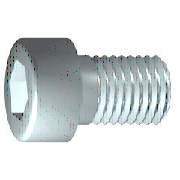
# Autodesk Inventor part: M3 x 5 - Socket Cap Screw - Standard (A2)
Saved by Autodesk Inventor 2016 SP1 (Build 200210100, 210)
## iProperties
Created: 2017-05-23
Part Number: M3 x 5 - Socket Cap Screw - Standard (A2)
Cost Center: P
Material: Stainless Steel
Description: Socket Cap Screw - Standard - (A2) - M3 x 5
Vendor: Generic Manufacturer
Document SubType Name: Modeling
Standard: ISO 4762
Designer: Matthew Lockham
Standard Revision: Fourth edition 2004-03-01
Standards Organization: ISO
Language: en-US
Size Designation: M3 x 5
Categories: <MemberInstance><Categories><Category DisplayName="Fasteners" InternalName="e4da775c-781d-43d5-af7c-5136215cf5a6" Mnemonic="FSTN"><Category DisplayName="Bolts" InternalName="536e6df0-f778-49ac-b2f2-25c71d2aa0b2" Mnemonic="SCRW"><CategoryParameter DisplayName="Nominal Diameter" InternalName="8bbe3f8e-44cf-40a9-a251-3a6edc8168d6" Mnemonic="nomdia"/><CategoryParameter DisplayName="Nominal Length" InternalName="238ecbaf-3e6c-45dd-aa95-4068c8e0fd02" Mnemonic="nomlen"/><CategoryParameter DisplayName="Thread Series Designation" InternalName="87c5849c-b3a5-4c3e-9c9b-2feecef9be86" Mnemonic="thrserdsgn"/><CategoryParameter DisplayName="Thread Class" InternalName="ebc0d23b-2cc6-4d2a-b376-d52aae53bab6" Mnemonic="thrclss"/><CategoryParameter DisplayName="Thread Designation" InternalName="586d5e89-370a-4089-914f-0110033585c7" Mnemonic="thrdesign"/><CategoryParameter DisplayName="Thread Type" InternalName="b4bbb7bc-d6aa-4c9f-a9a9-4152b9f6fe49" Mnemonic="thrtype"/><CategoryParameter DisplayName="Threads per Unit" InternalName="bdc6e7d2-ffd0-4d9c-a173-16b95ebb912d" Mnemonic="thrperunit1"/><CategoryParameter DisplayName="Thread Pitch" InternalName="bb82302e-82d8-4176-8fc1-c5d7bb17d5ad" Mnemonic="pitch1"/><CategoryParameter DisplayName="Nominal Diameter Designation" InternalName="03caf894-eafd-4c09-a035-916ac084b87b" Mnemonic="nomdiadesig"/><Category DisplayName="Socket Head" InternalName="55e06bf3-7e58-486c-bbdc-745fcc60664d" Mnemonic="CLSCRW"><CategoryParameter DisplayName="Shank Diameter" InternalName="179dbae3-102f-48bb-85fe-1e3ecd34f7cc" Mnemonic="grpdia"/><CategoryParameter DisplayName="Grip Length" InternalName="52eab69f-422f-4795-9995-175a1b827e67" Mnemonic="grplen"/><CategoryParameter DisplayName="Thread Length" InternalName="3268731d-5f9a-4750-8b01-4a959c46fbf2" Mnemonic="thrlen"/><CategoryParameter DisplayName="Head Diameter" InternalName="46177176-dbdd-4a1b-aefd-4c60c45016af" Mnemonic="headdia"/><CategoryParameter DisplayName="Head Height" InternalName="99c92c4c-4a02-4ebe-9e64-948fb169e19e" Mnemonic="headh"/><CategoryParameter DisplayName="Type" InternalName="59a7e495-7a0c-4a5c-bdfd-c090c5f6e2db" Mnemonic="type"/></Category></Category></Category><Category DisplayName="DataType" InternalName="23b78d0f-2648-40c6-8793-ca6db495c9e8" Mnemonic="DATATYPE"><CategoryParameter DisplayName="DisplayName" InternalName="05415f3d-3907-474b-a020-eb9d644f4cf3" Mnemonic="DISPLAYNAME"/><CategoryParameter DisplayName="InternalName" InternalName="cf1d0246-76d9-4b4a-8305-fa0409afb5c1" Mnemonic="INTERNALNAME"/><CategoryParameter DisplayName="Folder Name" InternalName="3f06958e-8713-4116-9be7-ed6184ecc97b" Mnemonic="FOLDERNAME"/><CategoryParameter DisplayName="Family Version" InternalName="914462f6-6e19-4b14-ba84-155b9680b1d0" Mnemonic="FAMILYREVISION"/><CategoryParameter DisplayName="ClipFormat" InternalName="bc51e27b-3422-4e78-93ef-cec197ddf230" Mnemonic="CLIPFORMAT"/><CategoryParameter DisplayName="IsMetric" InternalName="e2385c5b-1ea4-4823-96a8-8de651266ec3" Mnemonic="ISMETRIC"/><CategoryParameter DisplayName="Description" InternalName="13903e3d-64b1-4950-80da-f627842ea37f" Mnemonic="DESCRIPTION"/><CategoryParameter DisplayName="StdsOrg" InternalName="8f5914e1-4693-403f-8ab5-d37768198c9d" Mnemonic="STDSORG"/><CategoryParameter DisplayName="Standard" InternalName="0c0a119c-1e12-4c84-803f-101930972f5e" Mnemonic="STANDARD"/><CategoryParameter DisplayName="Manufacturer" InternalName="cd6c7a72-a28a-4e50-99a9-2c7f4e13e5ad" Mnemonic="MANUFACTURER"/><CategoryParameter DisplayName="Member Revision" InternalName="a65d44b9-392f-4f4f-857b-e4b3d54996fe" Mnemonic="MEMBERREVISION"/><CategoryParameter DisplayName="Standard Revision" InternalName="91d5a463-65c2-4fde-b823-3b7fea5e8e17" Mnemonic="STANDARDREVISION"/><CategoryParameter DisplayName="Revision Guid" InternalName="45a75005-10b1-4dfc-8d6d-dfe629f0b93c" Mnemonic="REVISIONGUID"/><CategoryParameter DisplayName="Designation" InternalName="2675968c-4ce5-49e0-a4f5-552d29089031" Mnemonic="DESIGNATION"/><CategoryParameter DisplayName="FileName" InternalName="8b46a4cc-9585-4fed-90c3-899f57e09a73" Mnemonic="FILENAME"/><CategoryParameter DisplayName="Default Row" InternalName="2af9ec52-faaa-4026-b378-f9fa4afca842" Mnemonic="DEFAULTROW"/><Category DisplayName="Part" InternalName="c0e0b642-3bcb-4cc8-9e80-f96d35c4afa4" Mnemonic="PART"><CategoryParameter DisplayName="Material" InternalName="818a152a-d3c3-49ca-80ee-df7d91421b8e" Mnemonic="MATERIAL"/><CategoryParameter DisplayName="Material Key" InternalName="5c9a8adb-dd2b-4535-b97f-0a94a95fe41f" Mnemonic="MATERIALKEY"/><CategoryParameter DisplayName="Part Number" InternalName="016b6077-bfbe-49bd-92c9-d8d59c39c941" Mnemonic="PARTNUMBER"/><CategoryParameter DisplayName="Stock Number" InternalName="4dba7c1c-e26c-444e-836c-b08b433409a8" Mnemonic="STOCKNUMBER"/></Category></Category></Categories><FamilyTemplate Id="si0145"><FamilyTemplateParameters><FamilyTemplateParameter ObjectType="kUserParameterObject" ValueType="xs:double" Id="1" ObjectReferenceKey="GUL"/><FamilyTemplateParameter ObjectType="kUserParameterObject" ValueType="xs:double" Id="2" ObjectReferenceKey="SPD"/><FamilyTemplateParameter ObjectType="kUserParameterObject" ValueType="xs:double" Id="3" ObjectReferenceKey="NLG"/><FamilyTemplateParameter ObjectType="kUserParameterObject" ValueType="xs:double" Id="4" ObjectReferenceKey="KOD"/><FamilyTemplateParameter ObjectType="kUserParameterObject" ValueType="xs:double" Id="5" ObjectReferenceKey="TOA"/><FamilyTemplateParameter ObjectType="kUserParameterObject" ValueType="xs:double" Id="6" ObjectReferenceKey="GD1"/><FamilyTemplateParameter ObjectType="kUserParameterObject" ValueType="xs:double" Id="7" ObjectReferenceKey="GEL"/><FamilyTemplateParameter ObjectType="kUserParameterObject" ValueType="xs:double" Id="8" ObjectReferenceKey="SW"/><FamilyTemplateParameter ObjectType="kUserParameterObject" ValueType="xs:double" Id="9" ObjectReferenceKey="THREADDIA"/><FamilyTemplateParameter ObjectType="kUserParameterObject" ValueType="xs:double" Id="10" ObjectReferenceKey="INTI"/><FamilyTemplateParameter ObjectType="kUserParameterObject" ValueType="xs:double" Id="11" ObjectReferenceKey="BDM"/><FamilyTemplateParameter ObjectType="kUserParameterObject" ValueType="xs:double" Id="12" ObjectReferenceKey="FAWI"/><FamilyTemplateParameter ObjectType="kUserParameterObject" ValueType="xs:double" Id="13" ObjectReferenceKey="RR"/><FamilyTemplateParameter ObjectType="kUserParameterObject" ValueType="xs:double" Id="14" ObjectReferenceKey="KOH"/><FamilyTemplateParameter ObjectType="kUserParameterObject" ValueType="xs:double" Id="15" ObjectReferenceKey="TPU"/><FamilyTemplateParameter ObjectType="kUserParameterObject" ValueType="xs:double" Id="16" ObjectReferenceKey="PTC"/><FamilyTemplateParameter ObjectType="kUserParameterObject" ValueType="xs:double" Id="17" ObjectReferenceKey="NND"/><FamilyTemplateParameter ObjectType="kUserParameterObject" ValueType="xs:double" Id="18" ObjectReferenceKey="GD"/><FamilyTemplateParameter ObjectType="kUserParameterObject" ValueType="xs:double" Id="19" ObjectReferenceKey="GAL"/><FamilyTemplateParameter ObjectType="kUserParameterObject" ValueType="xs:double" Id="20" ObjectReferenceKey="E0"/><FamilyTemplateParameter ObjectType="kPropertyObject" ValueType="xs:string" Id="100" ObjectReferenceKey="{32853F0F-3444-11d1-9E93-0060B03C1CA6}" SubObjectId="52"/><FamilyTemplateParameter ObjectType="kPropertyObject" ValueType="xs:string" Id="105" ObjectReferenceKey="{32853F0F-3444-11d1-9E93-0060B03C1CA6}" SubObjectId="5"/><FamilyTemplateParameter ObjectType="kPropertyObject" ValueType="xs:string" Id="106" ObjectReferenceKey="{32853F0F-3444-11d1-9E93-0060B03C1CA6}" SubObjectId="29"/><FamilyTemplateParameter ObjectType="kPartComponentDefinitionObject" ValueType="xs:string" Id="110" SubObjectId="Material"/><FamilyTemplateParameter ObjectType="kThreadFeatureObject" ValueType="xs:structure" Id="300" ObjectReferenceKey="1002000010000000a2070000000000008000000000000000" SubObjectId="ThreadInfo"><FamilyTemplateParameter ObjectType="" ValueType="xs:string" Id="301" SubObjectId="ThreadDesignation"/><FamilyTemplateParameter ObjectType="" ValueType="xs:string" Id="302" SubObjectId="ThreadType"/><FamilyTemplateParameter ObjectType="" ValueType="xs:string" Id="303" SubObjectId="ThreadClass"/></FamilyTemplateParameter><FamilyTemplateParameter ObjectType="kPropertyObject" ValueType="xs:string" Id="503" ObjectReferenceKey="{32853F0F-3444-11D1-9E93-0060B03C1CA6}" SubObjectId="9"/><FamilyTemplateParameter ObjectType="kPropertyObject" ValueType="xs:string" Id="504" ObjectReferenceKey="{32853F0F-3444-11D1-9E93-0060B03C1CA6}" SubObjectId="30"/><FamilyTemplateParameter ObjectType="kPartDocumentObject" ValueType="xs:string" Id="505" SubObjectId="DisplayName"/></FamilyTemplateParameters></FamilyTemplate><CategoryParameterMap><ParamToTemplateMap><ParamToTemplate CategoryParameter="//CategoryParameter[@InternalName='05415f3d-3907-474b-a020-eb9d644f4cf3']" ConstantValue="Socket Cap Screw"/><ParamToTemplate CategoryParameter="//CategoryParameter[@InternalName='cf1d0246-76d9-4b4a-8305-fa0409afb5c1']" ConstantValue="0228a834-b69c-46de-845a-346444175acc"/><ParamToTemplate CategoryParameter="//CategoryParameter[@InternalName='3f06958e-8713-4116-9be7-ed6184ecc97b']" ConstantValue="Socket Cap Screw"/><ParamToTemplate CategoryParameter="//CategoryParameter[@InternalName='914462f6-6e19-4b14-ba84-155b9680b1d0']" ConstantValue="10"/><ParamToTemplate CategoryParameter="//CategoryParameter[@InternalName='bc51e27b-3422-4e78-93ef-cec197ddf230']" ConstantValue="CF_INVENTOR.STDPARTS"/><ParamToTemplate CategoryParameter="//CategoryParameter[@InternalName='e2385c5b-1ea4-4823-96a8-8de651266ec3']" ConstantValue="true"/><ParamToTemplate CategoryParameter="//CategoryParameter[@InternalName='13903e3d-64b1-4950-80da-f627842ea37f']" ConstantValue="Hexagon Socket Head Cap Screw"/><ParamToTemplate CategoryParameter="//CategoryParameter[@InternalName='8f5914e1-4693-403f-8ab5-d37768198c9d']" ConstantValue="ISO"/><ParamToTemplate CategoryParameter="//CategoryParameter[@InternalName='0c0a119c-1e12-4c84-803f-101930972f5e']" ConstantValue="ISO 4762"/><ParamToTemplate CategoryParameter="//CategoryParameter[@InternalName='cd6c7a72-a28a-4e50-99a9-2c7f4e13e5ad']" TemplateParameter="104"/><ParamToTemplate CategoryParameter="//CategoryParameter[@InternalName='91d5a463-65c2-4fde-b823-3b7fea5e8e17']" ConstantValue="Fourth edition 2004-03-01"/><ParamToTemplate CategoryParameter="//CategoryParameter[@InternalName='45a75005-10b1-4dfc-8d6d-dfe629f0b93c']" ConstantValue="8a618e3f-b604-4408-b898-144709662ae0"/><ParamToTemplate CategoryParameter="//CategoryParameter[@InternalName='2af9ec52-faaa-4026-b378-f9fa4afca842']" ConstantValue="10"/><ParamToTemplate CategoryParameter="//CategoryParameter[@InternalName='a65d44b9-392f-4f4f-857b-e4b3d54996fe']" ConstantValue="69ce6232-463b-47b9-b677-461f109c7dae"/><ParamToTemplate CategoryParameter="//CategoryParameter[@InternalName='52eab69f-422f-4795-9995-175a1b827e67']" ConstantValue="1.25"/><ParamToTemplate CategoryParameter="//CategoryParameter[@InternalName='ebc0d23b-2cc6-4d2a-b376-d52aae53bab6']" ConstantValue="6g"/><ParamToTemplate CategoryParameter="//CategoryParameter[@InternalName='03caf894-eafd-4c09-a035-916ac084b87b']" ConstantValue="M3"/><ParamToTemplate CategoryParameter="//CategoryParameter[@InternalName='b4bbb7bc-d6aa-4c9f-a9a9-4152b9f6fe49']" ConstantValue="ISO Metric profile"/><ParamToTemplate CategoryParameter="//CategoryParameter[@InternalName='179dbae3-102f-48bb-85fe-1e3ecd34f7cc']" TemplateParameter="11"/><ParamToTemplate CategoryParameter="//CategoryParameter[@InternalName='2675968c-4ce5-49e0-a4f5-552d29089031']" TemplateParameter="100"/><ParamToTemplate CategoryParameter="//CategoryParameter[@InternalName='8b46a4cc-9585-4fed-90c3-899f57e09a73']" TemplateParameter="505"/><ParamToTemplate CategoryParameter="//CategoryParameter[@InternalName='3268731d-5f9a-4750-8b01-4a959c46fbf2']" TemplateParameter="7"/><ParamToTemplate CategoryParameter="//CategoryParameter[@InternalName='46177176-dbdd-4a1b-aefd-4c60c45016af']" TemplateParameter="4"/><ParamToTemplate CategoryParameter="//CategoryParameter[@InternalName='99c92c4c-4a02-4ebe-9e64-948fb169e19e']" TemplateParameter="14"/><ParamToTemplate CategoryParameter="//CategoryParameter[@InternalName='818a152a-d3c3-49ca-80ee-df7d91421b8e']" TemplateParameter="110"/><ParamToTemplate CategoryParameter="//CategoryParameter[@InternalName='238ecbaf-3e6c-45dd-aa95-4068c8e0fd02']" TemplateParameter="3"/><ParamToTemplate CategoryParameter="//CategoryParameter[@InternalName='8bbe3f8e-44cf-40a9-a251-3a6edc8168d6']" TemplateParameter="17"/><ParamToTemplate CategoryParameter="//CategoryParameter[@InternalName='016b6077-bfbe-49bd-92c9-d8d59c39c941']" TemplateParameter="105"/><ParamToTemplate CategoryParameter="//CategoryParameter[@InternalName='bb82302e-82d8-4176-8fc1-c5d7bb17d5ad']" TemplateParameter="16"/><ParamToTemplate CategoryParameter="//CategoryParameter[@InternalName='586d5e89-370a-4089-914f-0110033585c7']" TemplateParameter="301"/><ParamToTemplate CategoryParameter="//CategoryParameter[@InternalName='bdc6e7d2-ffd0-4d9c-a173-16b95ebb912d']" TemplateParameter="15"/></ParamToTemplateMap></CategoryParameterMap></MemberInstance>
Density: 8.08 g/cm^3
Appearance: Metal-Steel (Stainless, Brushed)
Saved_Yet: Not Saved
IsCustomPart: 0
Author: Matthew Lockham
Autodesk Inventor part; units mm, degrees
ref_plane "YZ Plane" through (0, 0, 0) normal (1, 0, 0) x (0, 1, 0)
ref_plane "XZ Plane" through (0, 0, 0) normal (0, 1, 0) x (-1, 0, 0)
ref_plane "XY Plane" through (0, 0, 0) normal (0, 0, 1) x (1, 0, 0)
sketch "Sketch1" plane through (0, 0, 0) normal (0, 0, 1) x (1, 0, 0)
  line L0 (-0.8667, 0) -> (5, 0)
  line L1 (5, 0) -> (5, 1.5)
  line L2 (5, 1.5) -> (1.25, 1.5)
  line L3 (1.25, 1.5) -> (0.9432, 1.5)
  line L4 (0.9432, 1.5) -> (0, 1.5)
  line L5 (0, 1.5) -> (0, 2.75)
  line L6 (0, 2.75) -> (-3, 2.75)
  line L7 (-3, 2.75) -> (-3, 1.4434)
  line L8 (-3, 1.4434) -> (-1.7, 1.4434)
  line L9 (-1.7, 1.4434) -> (-0.8667, 0)
  line L10 (-4.6, 0) -> (6.6, 0) projected
  line L11 (0, -0.55) -> (0, 3.3) projected
  line L12 (1.25, 1.5) -> (0, 1.5) construction
  dimension "d1" = 3.75
  dimension "d2" = 0.3068
  dimension "d3" = 3
  dimension "d4" = 1.3
  dimension "d5" = 60
  dimension "d6" = 3
  dimension "d7" = 3
  dimension "d8" = 2.8868
  dimension "d9" = 5.5
  dimension "d26" = 5
  constraints: 22 end point, 6 parallel, 2 collinear, 2 perpendicular, 1 horizontal, 1 point on line
  measures "d1" distance from line of L2.end L1
  measures "d2" distance of L3.end L2.end
  measures "d3" distance between parallel lines of L7 L5
  measures "d4" distance of L7.end L8.end
  measures "d5" angle of L9 L0
  measures "d6" diameter of L2 L0
  measures "d7" diameter of L4 L0
  measures "d8" diameter of L8 L0
  measures "d9" diameter of L6 L0
  measures "d26" distance between parallel lines of L11 L1
revolve "Body" add sketch "Sketch1" angle 360 about axis through (-0.8667, 0, 0) along (1, 0, 0)
sketch "Sketch2" plane through (-3, 0, 0) normal (-1, 0, 0) x (0, 0, 1)
  circle A0 centre (0, 0) radius 1.4434 projected
  line L0 (0, -3.85) -> (0, 3.85) projected
  line L1 (-3.85, 0) -> (3.85, 0) projected
  line L2 (1.4434, 0) -> (0.7217, -1.25)
  line L3 (0.7217, -1.25) -> (-0.7217, -1.25)
  line L4 (-0.7217, -1.25) -> (-1.4434, 0)
  line L5 (-1.4434, 0) -> (-0.7217, 1.25)
  line L6 (-0.7217, 1.25) -> (0.7217, 1.25)
  line L7 (0.7217, 1.25) -> (1.4434, 0)
  constraints: 12 end point, 1 coincident, 1 horizontal alignment, 1 point on line, 12 other
extrude "Slot" add sketch "Sketch2" against normal up to next contours L7 A0 | A0 L2 | L6 L0 A0 | A0 L0 L3 | L0 L6 A0 | A0 L3 L0 | L4 A0 | A0 L5
fillet "Fillet1" radius 0.3 1 edges at (-3, -2.75, 0)
thread "Thread" size "M3x0.5" class "6g" standard "ISO Metric Profile" length 3.75
chamfer "Chamfer1" distance 0.3067 distance2 0.3067 1 edges at (5, -1.5, 0) measured on face at (5, -1, 0)
ref_plane "Work Plane1" through (29, 0, 0) normal (0, -1, 0) x (1, 0, 0)
fillet "Fillet2" radius 0.1 1 edges at (0, -1.5, 0)
equation "\"d1\" = GEL"
equation "\"d3\" = KOH"
equation "\"d4\" = INTI"
equation "\"d6\" = GD"
equation "\"d7\" = BDM"
equation "\"d8\" = 1.1547 * SW"
equation "\"d9\" = KOD"
equation "\"d26\" = NLG"
equation "\"d30\" = R"
equation "\"d17\" = RR"
equation "\"d13\" = GEL"
equation "\"d15\" = -0.5 * SPD + 0.5 * GD"
equation "\"d16\" = GUL"
equation "\"GD\" = 3"
equation "\"NLG\" = 5"
equation "\"GEL\" = 3.75"
equation "\"KOD\" = 5.5"
equation "\"KOH\" = 3"
equation "\"INTI\" = 1.3"
equation "\"GAL\" = 0.61345 * PTC"
equation "\"GUL\" = 0.61345 * PTC"
equation "\"BDM\" = NND"
equation "\"SW\" = 2.5"
equation "\"RR\" = 0.3"
equation "\"SPD\" = NND - 1.2269 * PTC"
equation "\"R\" = 0.1"
equation "\"TOA\" = 30deg"
equation "\"GD1\" = THREADDIA - 1.2269 * PTC"
equation "\"THREADDIA\" = 3"
equation "\"FAWI\" = 45deg"
equation "\"PTC\" = 0.5"
equation "\"NND\" = 3"
equation "\"E0\" = 1.155 * SW"
body "Solid1"
